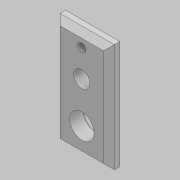
# Autodesk Inventor part: exercise2-1
Saved by Autodesk Inventor 2018 (Build 220112000, 112)
## iProperties
Created: 2020-09-19
Part Number: exercise2-1
Material: 一般
Document SubType Name: Modeling
Designer: 王鼎鈞
Density: 1 g/cm^3
Appearance: 預設
Author: 王鼎鈞
Autodesk Inventor part; units mm, degrees
ref_plane "YZ Plane" through (0, 0, 0) normal (1, 0, 0) x (0, 1, 0)
ref_plane "XZ Plane" through (0, 0, 0) normal (0, 1, 0) x (-1, 0, 0)
ref_plane "XY Plane" through (0, 0, 0) normal (0, 0, 1) x (1, 0, 0)
sketch "草圖1" plane through (0, 0, 0) normal (1, 0, 0) x (0, 1, 0)
  line L0 (-6, 0) -> (36, 0) projected
  line L1 (0, -240) -> (0, 40) projected
  line L2 (0, 0) -> (30, 0)
  line L3 (30, 0) -> (30, -200)
  line L4 (30, -200) -> (0, -200)
  line L5 (0, -200) -> (0, 0)
  dimension "d0" = 30
  dimension "d1" = 200
  constraints: 8 end point, 2 parallel, 1 horizontal, 1 perpendicular
  measures "d0" distance of L3.end L4.end
  measures "d1" distance of L2.end L3.end
extrude "擠出1" add sketch "草圖1" along normal mid plane 100
chamfer "倒角1" distance 10 angle 45 8 edges at (50, 30, -100) (0, 30, 0) (-50, 30, -100) (0, 30, -200) (50, 0, -100) (0, 0, 0) (0, 0, -200) (-50, 0, -100)
sketch "草圖2" plane through (-40, 30, -190) normal (0, 1, 0) x (1, 0, 0)
  line L0 (40, -190) -> (40, 28.9539)
  line L1 (-10, -190) -> (90, -190) projected
  circle A0 centre (40, -165) radius 7.5
  circle A1 centre (40, -115) radius 15
  circle A2 centre (40, -40) radius 22.5
  point P0 (40, -90.6326)
  point P1 (40, -37.7519)
  dimension "d7" = 25
  dimension "d8" = 15
  dimension "d9" = 30
  dimension "d10" = 45
  dimension "d11" = 50
  dimension "d12" = 75
  constraints: 5 point on line, 3 centre point, 2 end point, 1 coincident, 1 vertical
  measures "d7" distance from line of L1 point (40, -165)
  measures "d8" diameter of A0
  measures "d9" diameter of A1
  measures "d10" diameter of A2
  measures "d11" distance of A0.centre A1.centre
  measures "d12" distance of A1.centre A2.centre
extrude "擠出2" cut sketch "草圖2" against normal blind 108
chamfer "倒角2" distance 5 angle 45 3 edges at (-15, 30, -75) (-7.5, 30, -25) (-22.5, 30, -150)
